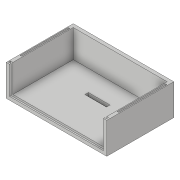
# Autodesk Inventor part: Sharp 2Y0A02 Case
Saved by Autodesk Inventor 2018.3 (Build 223284000, 284)
## iProperties
Created: 2018-12-13
Part Number: Sharp 2Y0A02 Case
Material: Generic
Document SubType Name: Modeling
Designer: aye06091
Mass: 4.50808 g
Surface Area: 66.9433 cm^2
Volume: 4.50808 cm^3
Density: 1 g/cm^3
Appearance: Default
Author: aye06091
Autodesk Inventor part; units mm, degrees
ref_plane "YZ Plane" through (0, 0, 0) normal (1, 0, 0) x (0, 1, 0)
ref_plane "XZ Plane" through (0, 0, 0) normal (0, 1, 0) x (-1, 0, 0)
ref_plane "XY Plane" through (0, 0, 0) normal (0, 0, 1) x (1, 0, 0)
sketch "Sketch1" plane through (0, 0, 0) normal (0, 0, 1) x (1, 0, 0)
  line L0 (47.9298, -1.5875) -> (47.9298, -16.4338)
  line L1 (47.9298, -16.4338) -> (0, -16.4338)
  line L2 (0, -16.4338) -> (0, -1.5875)
  line L3 (1.5875, -1.5875) -> (46.3423, -1.5875)
  line L4 (46.3423, -1.5875) -> (46.3423, -14.8463)
  line L5 (46.3423, -14.8463) -> (1.5875, -14.8463)
  line L6 (1.5875, -14.8463) -> (1.5875, -1.5875)
  line L7 (1.5875, -1.5875) -> (0, -1.5875)
  line L8 (46.3423, -1.5875) -> (47.9298, -1.5875)
  line L9 (0, 0) -> (1.5875, 0)
  line L10 (46.3423, 0) -> (47.9298, 0)
  dimension "d0" = 47.9298
  dimension "d1" = 16.4338
  dimension "d2" = 44.7548
  dimension "d4" = 13.2588
  dimension "d12" = 1.5875
  constraints: 22 end point, 5 parallel, 4 perpendicular, 3 horizontal, 3 point on line
  measures "d0" distance of L9.start L10.end
  measures "d1" distance of L1.end L9.start
  measures "d2" distance of L3.start L3.end
  measures "d4" distance of L5.end L3.start
  measures "d12" distance between parallel lines of L2 L6
extrude "Extrusion1" add sketch "Sketch1" against normal blind 25.4 contours L0 L1 L2 L7 L6 L5 L4 L8
sketch "Sketch2" plane through (1.5875, -14.8463, 0) normal (0, 1, 0) x (1, 0, 0)
  line L0 (44.7548, 0) -> (44.7548, 25.4) projected
  line L1 (0, 0) -> (0, 25.4) projected
  line L2 (0.127, 25.4) -> (44.6278, 25.4)
  line L3 (44.6278, 25.4) -> (44.6278, 0)
  line L4 (44.6278, 0) -> (0.127, 0)
  line L5 (0.127, 0) -> (0.127, 25.4)
  line L6 (17.1958, 15.4178) -> (27.559, 15.4178)
  line L7 (27.559, 15.4178) -> (27.559, 13.716)
  line L8 (27.559, 13.716) -> (17.1958, 13.716)
  line L9 (17.1958, 13.716) -> (17.1958, 15.4178)
  point P0 (-1.5875, 0)
  dimension "d10" = 44.5008
  dimension "d13" = 0.127
  dimension "d14" = 0.127
  dimension "d15" = 10.3632
  dimension "d16" = 1.7018
  dimension "d17" = 17.0688
  dimension "d18" = 17.0688
  dimension "d22" = 25.4
  dimension "d23" = 9.9822
  constraints: 16 end point, 4 parallel, 2 horizontal, 2 perpendicular, 1 point on line
  measures "d10" distance between parallel lines of L3 L5
  measures "d13" distance between parallel lines of L1 L5
  measures "d14" distance between parallel lines of L0 L3
  measures "d15" distance of L6.start L6.end
  measures "d16" distance of L6.end L7.end
  measures "d17" distance between parallel lines of L5 L9
  measures "d18" distance between parallel lines of L3 L7
  measures "d22" distance of L4.end L2.start
  measures "d23" distance between parallel lines of L2 L6
extrude "Extrusion2" cut sketch "Sketch2" against normal blind 25.4 contours L6 L7 L8 L9
sketch "Sketch3" plane through (0, -1.5875, 0) normal (0, 1, 0) x (1, 0, 0)
  line L0 (1.5875, 0) -> (0, 0) projected
  line L1 (1.5875, 0) -> (1.5875, 25.4) projected
  line L2 (0, 0) -> (0, 25.4) projected
  line L3 (0.3969, 1.27) -> (1.1906, 1.27)
  line L4 (1.1906, 1.27) -> (1.1906, 24.13)
  line L5 (1.1906, 24.13) -> (0.3969, 24.13)
  line L6 (0.3969, 24.13) -> (0.3969, 1.27)
  line L7 (46.7392, 1.27) -> (47.5329, 1.27)
  line L8 (47.5329, 1.27) -> (47.5329, 24.13)
  line L9 (47.5329, 24.13) -> (46.7392, 24.13)
  line L10 (46.7392, 24.13) -> (46.7392, 1.27)
  line L11 (46.3423, 0) -> (1.5875, 0) projected
  line L12 (47.9298, 0) -> (47.9298, 25.4) projected
  dimension "d26" = 22.86
  dimension "d27" = 1.27
  dimension "d28" = 0.3969
  dimension "d29" = 0.7937
  dimension "d30" = 0.3969
  dimension "d31" = 0.7937
  dimension "d32" = 1.27
  dimension "d33" = 0.3969
  constraints: 16 end point, 4 parallel, 2 horizontal, 2 perpendicular, 2 point on line
  measures "d26" distance of L5.end L3.start
  measures "d27" distance between parallel lines of L0 L3
  measures "d28" distance between parallel lines of L2 L6
  measures "d29" distance of L3.start L3.end
  measures "d30" distance between parallel lines of L1 L4
  measures "d31" distance of L7.start L7.end
  measures "d32" distance between parallel lines of L11 L7
  measures "d33" distance between parallel lines of L12 L8
extrude "Extrusion3" cut sketch "Sketch3" against normal blind 3.175
sketch "Sketch4" plane through (0, 0, -25.4) normal (0, 0, -1) x (-1, 0, 0)
  line L0 (-47.9298, -1.5875) -> (-47.9298, -16.4338) projected
  line L1 (-47.9298, -16.4338) -> (0, -16.4338) projected
  line L2 (-47.9298, -1.5875) -> (0, -1.5875)
  line L3 (0, -1.5875) -> (0, -16.4338)
  line L4 (0, -16.4338) -> (-47.9298, -16.4338)
  line L5 (-47.9298, -16.4338) -> (-47.9298, -1.5875)
  point P0 (0, 0)
  constraints: 8 end point, 2 parallel, 1 horizontal, 1 perpendicular
extrude "Extrusion4" add sketch "Sketch4" along normal blind 1.5875
sketch "Sketch5" plane through (0, 0, 0) normal (0, 0, 1) x (1, 0, 0)
  line L0 (47.9298, -16.4338) -> (47.9298, -1.5875) projected
  line L1 (47.9298, -1.5875) -> (46.3423, -1.5875) projected
  line L2 (46.3423, -1.5875) -> (46.3423, -14.8463) projected
  line L3 (46.3423, -14.8463) -> (1.5875, -14.8463) projected
  line L4 (1.5875, -14.8463) -> (1.5875, -1.5875) projected
  line L5 (1.5875, -1.5875) -> (0, -1.5875) projected
  line L6 (0, -1.5875) -> (47.9298, -1.5875)
  line L7 (47.9298, -1.5875) -> (47.9298, -16.4338)
  line L8 (47.9298, -16.4338) -> (0, -16.4338)
  line L9 (0, -16.4338) -> (0, -1.5875)
  point P0 (0, 0)
  constraints: 8 end point, 2 parallel, 1 horizontal, 1 perpendicular
extrude "Extrusion5" add sketch "Sketch5" along normal blind 4.9657 contours L8 L9 L5 L4 L3 L2 L1 L0
sketch "Sketch6" plane through (1.5875, -1.5875, -25.4) normal (0, 1, 0) x (1, 0, 0)
  line L0 (-1.1807, -29.6799) -> (45.561, -29.6799)
  line L1 (45.561, -29.6799) -> (45.561, -28.7782)
  line L2 (45.561, -28.7782) -> (-1.1807, -28.7782)
  line L3 (-1.1807, -28.7782) -> (-1.1807, -29.6799)
  line L4 (0, -30.3657) -> (-1.5875, -30.3657) projected
  point P0 (-1.5875, -25.4)
  dimension "d42" = 0.9017
  dimension "d43" = 0.6858
  constraints: 8 end point, 2 parallel, 1 horizontal, 1 perpendicular
  measures "d42" distance between parallel lines of L2 L0
  measures "d43" distance between parallel lines of L4 L0
extrude "Extrusion6" cut sketch "Sketch6" against normal blind 14.2875
body "Solid1"
